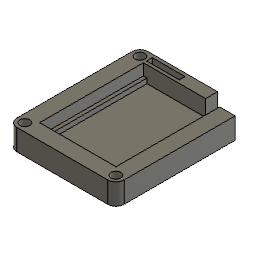
Mini Arcade Game Case Top (Autodesk Fusion 360 archive; units mm, degrees)
design "Mini Arcade Game Case"
part number: 2026-02-18-05-45-24-151
Autodesk Fusion 360 part; units mm, degrees
sketch "Sketch1" plane through (0, 0, 0) normal (0, 1, 0) x (1, 0, 0)
  line L0 (0, 0) -> (65.7, 0)
  line L1 (65.7, 0) -> (65.7, 80.4)
  line L2 (65.7, 80.4) -> (0, 80.4)
  line L3 (0, 80.4) -> (0, 0)
  line L4 (9.5, 73) -> (56.2, 73)
  line L5 (56.2, 73) -> (56.2, 9.5)
  line L6 (56.2, 9.5) -> (9.5, 9.5)
  line L7 (9.5, 9.5) -> (9.5, 73)
  line L8 (54.7, 80.4) -> (46, 80.4)
  line L9 (9.5, 78.4) -> (29.5, 78.4)
  line L10 (29.5, 78.4) -> (29.5, 74.9)
  line L11 (29.5, 74.9) -> (9.5, 74.9)
  line L12 (9.5, 74.9) -> (9.5, 78.4)
  line L13 (65.7, 80.4) -> (47.5, 80.4)
  line L14 (47.5, 80.4) -> (47.5, 73)
  line L15 (47.5, 73) -> (65.7, 73)
  line L16 (65.7, 73) -> (65.7, 80.4)
  circle A0 centre (5, 5) radius 1.7
  circle A1 centre (5, 5) radius 3
  circle A2 centre (60.7, 5) radius 1.7
  circle A3 centre (60.7, 5) radius 3
  circle A4 centre (5, 75.4) radius 1.7
  circle A5 centre (5, 75.4) radius 3
  line L17 (11.7, 73) -> (53.9, 73)
  line L18 (53.9, 73) -> (53.9, 9.5)
  line L19 (53.9, 9.5) -> (11.7, 9.5)
  line L20 (11.7, 9.5) -> (11.7, 73)
  dimension "d1" = 65.7
  dimension "d2" = 80.4
  dimension "d3" = 46.7
  dimension "d5" = 9.5
  dimension "d6" = 9.5
  dimension "d31" = 20
  dimension "d32" = 3.5
  dimension "d33" = 9.5
  dimension "d40" = 18.2
  dimension "d43" = 7.4
  dimension "d44" = 3.4
  dimension "d45" = 6
  dimension "d46" = 2
  dimension "d47" = 5
  dimension "d48" = 5
  dimension "d49" = 3.4
  dimension "d50" = 5
  dimension "d51" = 5
  dimension "d52" = 6
  dimension "d53" = 3.4
  dimension "d54" = 5
  dimension "d55" = 5
  dimension "d56" = 6
  dimension "d57" = 42.2
  dimension "d58" = 2.2
  dimension "d59" = 63.5
  dimension "d60" = 63.5
  constraint horizontal L0
  constraint vertical L1
  constraint horizontal L2
  constraint vertical L3
  constraint coincident L0.start L3.end
  constraint horizontal L4
  constraint vertical L5
  constraint horizontal L6
  constraint vertical L7
  constraint horizontal L8
  constraint coincident L2 L8.start
  constraint horizontal L9
  constraint vertical L10
  constraint horizontal L11
  constraint vertical L12
  constraint horizontal L13
  constraint vertical L14
  constraint horizontal L15
  constraint vertical L16
  constraint concentric A0 A1
  constraint concentric A2 A3
  constraint concentric A4 A5
  constraint horizontal L17
  constraint vertical L18
  constraint horizontal L19
  constraint vertical L20
  constraint coincident L4 L17.start
  measures "d1" distance of L0.start L0.end
  measures "d2" distance of L0.start L2.end
  measures "d3" distance of L4.start L4.end
  measures "d5" distance of L1 L5
  measures "d6" distance of L0 L6
  measures "d31" distance of L9.start L9.end
  measures "d32" distance of L9.start L11.end
  measures "d33" distance of L3 L12
  measures "d40" distance of L1.end L13.end
  measures "d43" distance of L8.start L15
  measures "d44" diameter of A0
  measures "d45" diameter of A1
  measures "d46" distance of L2 L9
  measures "d47" distance of L0 A0.centre
  measures "d48" distance of L3 A0.centre
  measures "d49" diameter of A2
  measures "d50" distance of L0 A2.centre
  measures "d51" distance of L1 A2.centre
  measures "d52" diameter of A3
  measures "d53" diameter of A4
  measures "d54" distance of L2 A4.centre
  measures "d55" distance of L3 A4.centre
  measures "d56" diameter of A5
  measures "d57" distance of L17.start L17.end
  measures "d58" distance of L7 L20
  measures "d59" distance of L4 L6
  measures "d60" distance of L17 L19
extrude "Extrude4" add sketch "Sketch1" against normal blind 3 contours L0 L1 L2 L3 L4 L5 L6 L7 L8 L14 L15 L17 L19 | L4 L5 L6 L15 L18 | L4 L6 L15 L17 L18 L19 L20 | L4 L6 L7 L20 | A1 | A3 | A5
extrude "Extrude6" add sketch "Sketch1" along normal blind 3 contours L4 L5 L6 L15 L18 | L4 L6 L7 L20 | A1 | A3 | A5
extrude "Extrude5" add sketch "Sketch1" along normal blind 10 contours L0 L1 L2 L3 L4 L5 L6 L7 L8 L14 L15 L17 L19
fillet "Fillet1" radius 5 3 edges at (65.7, 3.5, 0) (0, 3.5, 0) (0, 3.5, -80.4)

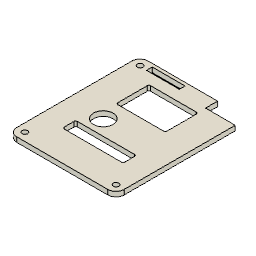
design "Mini Arcade Game Bottom"
part number: 2026-03-19-11-16-55-679
Autodesk Fusion 360 part; units mm, degrees
sketch "Sketch1" plane through (0, 0, 0) normal (0, 1, 0) x (1, 0, 0)
  line L0 (0, 0) -> (65.7, 0)
  line L1 (65.7, 0) -> (65.7, 80.4)
  line L2 (65.7, 80.4) -> (0, 80.4)
  line L3 (0, 80.4) -> (0, 0)
  circle A0 centre (5, 5) radius 1.7
  circle A1 centre (60.7, 5) radius 1.7
  circle A2 centre (5, 75.4) radius 1.7
  line L4 (65.7, 80.4) -> (47.5, 80.4)
  line L5 (47.5, 80.4) -> (47.5, 73)
  line L6 (47.5, 73) -> (65.7, 73)
  line L7 (65.7, 73) -> (65.7, 80.4)
  line L8 (9.5, 78.4) -> (29.5, 78.4)
  line L9 (29.5, 78.4) -> (29.5, 74.9)
  line L10 (29.5, 74.9) -> (9.5, 74.9)
  line L11 (9.5, 74.9) -> (9.5, 78.4)
  line L12 (14.35, 26.7) -> (51.35, 26.7)
  line L13 (51.35, 26.7) -> (51.35, 18.7)
  line L14 (51.35, 18.7) -> (14.35, 18.7)
  line L15 (14.35, 18.7) -> (14.35, 26.7)
  line L16 (17.85, 68) -> (47.85, 68)
  line L17 (47.85, 68) -> (47.85, 48)
  line L18 (47.85, 48) -> (17.85, 48)
  line L19 (17.85, 48) -> (17.85, 68)
  circle A3 centre (21.91, 36.02) radius 6
  dimension "d1" = 65.7
  dimension "d2" = 80.4
  dimension "d3" = 3.4
  dimension "d4" = 5
  dimension "d5" = 5
  dimension "d7" = 3.4
  dimension "d8" = 5
  dimension "d9" = 5
  dimension "d11" = 3.4
  dimension "d12" = 5
  dimension "d13" = 5
  dimension "d15" = 18.2
  dimension "d16" = 7.4
  dimension "d17" = 20
  dimension "d18" = 3.5
  dimension "d19" = 2
  dimension "d20" = 9.5
  dimension "d27" = 37
  dimension "d28" = 8
  dimension "d30" = 30
  dimension "d31" = 20
  dimension "d34" = 12
  dimension "d36" = 9.32
  dimension "d43" = 17.85
  constraint horizontal L0
  constraint vertical L1
  constraint horizontal L2
  constraint vertical L3
  constraint coincident L0.start L3.end
  constraint horizontal L4
  constraint vertical L5
  constraint horizontal L6
  constraint vertical L7
  constraint horizontal L8
  constraint vertical L9
  constraint horizontal L10
  constraint vertical L11
  constraint horizontal L12
  constraint vertical L13
  constraint horizontal L14
  constraint vertical L15
  constraint horizontal L16
  constraint vertical L17
  constraint horizontal L18
  constraint vertical L19
  measures "d1" distance of L0.start L0.end
  measures "d2" distance of L0.start L2.end
  measures "d3" diameter of A0
  measures "d4" distance of L0 A0.centre
  measures "d5" distance of L3 A0.centre
  measures "d7" diameter of A1
  measures "d8" distance of L0 A1.centre
  measures "d9" distance of L1 A1.centre
  measures "d11" diameter of A2
  measures "d12" distance of L2 A2.centre
  measures "d13" distance of L3 A2.centre
  measures "d15" distance of L1.end L4.end
  measures "d16" distance of L1.end L6.end
  measures "d17" distance of L8.start L8.end
  measures "d18" distance of L8.start L10.end
  measures "d19" distance of L2 L8
  measures "d20" distance of L3 L11
  measures "d27" distance of L12.start L12.end
  measures "d28" distance of L12.start L14.end
  measures "d30" distance of L16.start L16.end
  measures "d31" distance of L16.start L18.end
  measures "d34" diameter of A3
  measures "d36" distance of L12 A3.centre
  measures "d43" distance of L3 L19
extrude "Extrude1" add sketch "Sketch1" along normal blind 3 contours L0 L1 L2 L3 L5 L6
fillet "Fillet1" radius 5 3 edges at (65.7, 1.5, 0) (0, 1.5, 0) (0, 1.5, -80.4)
fillet "Fillet2" radius 1 8 edges at (17.85, 1.5, -68) (14.35, 1.5, -26.7) (47.85, 1.5, -68) (51.35, 1.5, -26.7) (51.35, 1.5, -18.7) (47.85, 1.5, -48) (17.85, 1.5, -48) (14.35, 1.5, -18.7)
